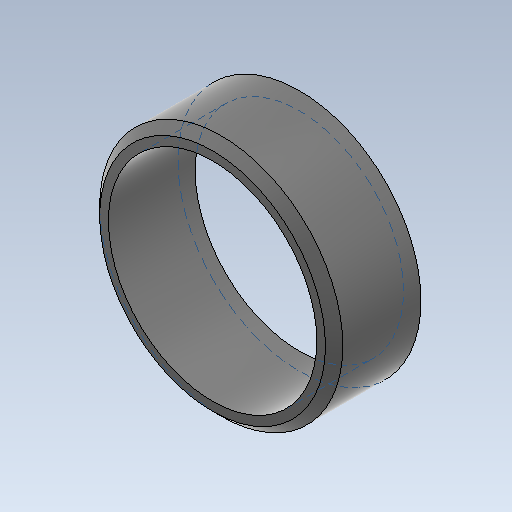
# Autodesk Inventor part: オイレスw5f10-12n
Saved by Autodesk Inventor 2020 (Build 240168000, 168)
## iProperties
Created: 2020-02-11
Part Number: オイレスw5f10-12n
Material: アセタール樹脂、黒
Document SubType Name: Modeling
Designer: happy
Density: 1.425 g/cm^3
Appearance: 滑らか - 黒
Mass: 0.283342 g
Surface Area: 4.76881 cm^2
Volume: 0.198837 cm^3
Author: happy
Autodesk Inventor part; units mm, degrees
ref_plane "YZ Plane" through (0, 0, 0) normal (1, 0, 0) x (0, 1, 0)
ref_plane "XZ Plane" through (0, 0, 0) normal (0, 1, 0) x (-1, 0, 0)
ref_plane "XY Plane" through (0, 0, 0) normal (0, 0, 1) x (1, 0, 0)
sketch "スケッチ1" plane through (0, 0, 0) normal (0, 0, 1) x (1, 0, 0)
  circle A0 centre (0, 0) radius 7
  circle A1 centre (0, 0) radius 6
  dimension "d0" = 14
  dimension "d1" = 12
  constraints: 2 centre point, 2 coincident
  measures "d0" diameter of A0
  measures "d1" diameter of A1
extrude "押し出し1" add sketch "スケッチ1" along normal blind 5
chamfer "面取り1" distance 0.5 angle 45 1 edges at (-7, 0, 5)
